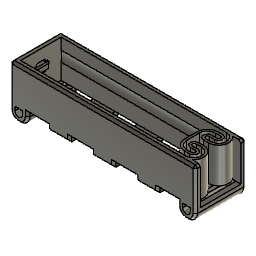
porta_pila_reforzado v2 (Autodesk Fusion 360 design; units mm, degrees)
Autodesk Fusion 360 part; units mm, degrees
note: some values were not read from the file. Set by a fixed rule: which face or edge a step refers to.
sketch "Sketch1" plane through (0, 0, 0) normal (0, 0, 1) x (1, 0, 0)
  line L0 (42, -11.5) -> (-42, -11.5)
  line L1 (-42, -11.5) -> (-42, 11.5)
  line L2 (-42, 11.5) -> (42, 11.5)
  line L3 (42, 11.5) -> (42, -11.5)
  line L4 (42, -11.5) -> (-42, 11.5) construction
  line L5 (-42, -11.5) -> (42, 11.5) construction
  dimension "d1" = 23
  dimension "d2" = 84
  constraint perpendicular L0 L1
  constraint parallel L0 L2
  constraint parallel L1 L3
  constraint horizontal L0
  constraint coincident L4 origin
  constraint coincident L5 origin
  measures "d1" distance of L0.end L1.end
  measures "d2" distance of L1.end L2.end
  measures "d8" distance of L0.start
extrude "Extrude1" add sketch "Sketch1" along normal blind 17
sketch "Sketch2" plane through (0, 0, 17) normal (0, 0, 1) x (-1, 0, 0)
  line L0 (-42, -11.5) -> (42, -11.5)
  line L1 (42, -11.5) -> (42, 11.5)
  line L2 (42, 11.5) -> (-42, 11.5)
  line L3 (-42, 11.5) -> (-42, -11.5)
  line L4 (39.5, -9.2) -> (-28.5, -9.2)
  line L5 (-28.5, -9.2) -> (-28.5, 9.2)
  line L6 (-28.5, 9.2) -> (39.5, 9.2)
  line L7 (39.5, 9.2) -> (39.5, -9.2)
  line L8 (42, 0) -> (39.5, 0) construction
  dimension "d5" = 68
  dimension "d6" = 18.4
  dimension "d7" = 2.5
  dimension "d8" = 1.8
  constraint horizontal L4
  constraint vertical L5
  constraint horizontal L6
  constraint vertical L7
  constraint midpoint L1 L8.start
  constraint midpoint L7 L8.end
  constraint horizontal L8
  measures "d5" distance of L4.start L4.end
  measures "d6" distance of L4.start L6.end
  measures "d7" distance of L1 L7
extrude "Extrude2" cut sketch "Sketch2" against normal through all contours L4 L5 L6 L7
sketch "Sketch3" plane through (28.5, 0, 0) normal (-1, 0, 0) x (0, -1, 0)
  line L0 (-9.2, 0) -> (9.2, 0)
  line L1 (9.2, 0) -> (9.2, 17)
  line L2 (9.2, 17) -> (-9.2, 17)
  line L3 (-9.2, 17) -> (-9.2, 0)
  circle A0 centre (0, 9.5) radius 9.5
  dimension "d10" = 19
  constraint coincident origin A0
  constraint vertical origin A0.centre
  measures "d10" diameter of A0
extrude "Extrude3" cut sketch "Sketch3" along normal blind 68 contours L3 A0 | L1 A0
sketch "Sketch4" plane through (0, 0, 17) normal (0, 0, 1) x (-1, 0, 0)
  line L0 (39.5, 9.2) -> (39.5, -9.2)
  line L1 (39.5, -9.2) -> (-28.5, -9.2)
  line L2 (-28.5, -9.2) -> (-28.5, 9.2)
  line L3 (-28.5, 9.2) -> (39.5, 9.2)
  line L4 (-42, -11.5) -> (42, -11.5)
  line L5 (42, -11.5) -> (42, 11.5)
  line L6 (42, 11.5) -> (-42, 11.5)
  line L7 (-42, 11.5) -> (-42, -11.5)
  line L8 (-28.5, 2.95) -> (-28.5, -2.95)
  arc A0 (-33.05, -7.5) -> (-28.5, -2.95) centre (-33.05, -2.95) ccw
  line L9 (-33.05, -7.5) -> (-35.45, -7.5)
  arc A1 (-35.45, -3.8) -> (-35.45, -7.5) centre (-35.45, -5.65) ccw
  line L10 (-35.45, -3.8) -> (-33.05, -3.8)
  arc A2 (-33.05, -3.8) -> (-33.05, -2.1) centre (-33.05, -2.95) ccw
  line L11 (-33.05, -2.1) -> (-35.45, -2.1)
  arc A3 (-35.45, -2.1) -> (-35.45, -9.2) centre (-35.45, -5.65) ccw
  line L12 (-35.45, -9.2) -> (-28.5, -9.2)
  line L13 (-35.45, -10.2) -> (-28.5, -10.2)
  arc A4 (-35.45, -1.1) -> (-35.45, -10.2) centre (-35.45, -5.65) ccw
  line L14 (-33.05, -1.1) -> (-35.45, -1.1)
  arc A5 (-33.05, -4.8) -> (-33.05, -1.1) centre (-33.05, -2.95) ccw
  line L15 (-35.45, -4.8) -> (-33.05, -4.8)
  arc A6 (-35.45, -4.8) -> (-35.45, -6.5) centre (-35.45, -5.65) ccw
  line L16 (-33.05, -6.5) -> (-35.45, -6.5)
  arc A7 (-33.05, -6.5) -> (-29.5, -2.95) centre (-33.05, -2.95) ccw
  line L17 (-29.5, 2.95) -> (-29.5, -2.95)
  line L18 (-39, -11.5) -> (-39, 11.5) construction
  line L19 (-28.5, 0) -> (-42, 0)
  line L20 (-28.5, -9.2) -> (-28.5, -10.2)
  line L21 (-29.5, 2.95) -> (-28.5, 2.95)
  line L22 (-35.45, -10.2) -> (-42, -10.2)
  line L23 (-35.45, -9.2) -> (-42, -9.2)
  dimension "d14" = 3
  dimension "d20" = 1.7
  dimension "d21" = 1.7
  dimension "d22" = 1.5
  dimension "d23" = 1
  constraint tangent L8 A0
  constraint tangent A0 L9
  constraint tangent L9 A1
  constraint tangent A1 L10
  constraint tangent L10 A2
  constraint horizontal L11
  constraint tangent L11 A3
  constraint coincident L1.end L2.start
  constraint coincident A1.centre A3.centre
  constraint midpoint L2 L8
  constraint tangent A2 L11
  constraint tangent A3 L12
  constraint horizontal L12
  constraint horizontal L9
  constraint horizontal L10
  constraint coincident L4 L18.start
  constraint coincident L6 L18.end
  constraint perpendicular L6 L18
  constraint tangent A3 L18
  constraint parallel L12 L13
  constraint concentric A3 A4
  constraint parallel L11 L14
  constraint concentric A2 A5
  constraint parallel L10 L15
  constraint concentric A1 A6
  constraint parallel L9 L16
  constraint concentric A0 A7
  constraint parallel L8 L17
  constraint tangent L16 A7
  constraint tangent L13 A4
  constraint tangent L15 A6
  constraint tangent A4 L14
  constraint tangent L14 A5
  constraint tangent A5 L15
  constraint tangent A6 L16
  constraint tangent A7 L17
  constraint vertical L8
  constraint coincident A0.centre A2.centre
  constraint midpoint L8 L19.start
  constraint midpoint L7 L19.end
  constraint perpendicular L13 L20
  constraint horizontal L21
  constraint coincident L7 L22.end
  constraint tangent A4 L22
  constraint coincident L7 L23.end
  constraint tangent A3 L23
  measures "d14" distance of L7 L18
  measures "d20" distance of L9 L12
  measures "d21" distance of L15 L16
  measures "d23" distance of L12 L13
extrude "Extrude4" cut sketch "Sketch4" against normal through all contours L2 A0 L9 A1 L10 A2 L11 A3 L12 | L7 A4 L14 A5 L15 A6 L16 A7 L17 L19 L23
mirror "Mirror1" about plane through (0, 0, 0) normal (0, 1, 0) of "Extrude4"
extrude "Extrude5" cut 2 faces at (28.5, 9.2749, 9.8979) (28.5, -9.2749, 9.1021) along direction (1, 0, 0) blind 7.95
sketch "Sketch5" plane through (0, -11.5, 0) normal (0, -1, 0) x (1, 0, 0)
  line L0 (-42, 0) -> (42, 0)
  line L1 (42, 0) -> (42, 17)
  line L2 (42, 17) -> (-42, 17)
  line L3 (-42, 17) -> (-42, 0)
  circle A0 centre (-38, -1.7) radius 1.7
  circle A1 centre (38, -1.7) radius 1.7
  line L4 (-42, 0) -> (-42, -1.7)
  arc A2 (-42, -1.7) -> (-34, -1.7) centre (-38, -1.7) ccw
  line L5 (-34, -1.7) -> (-34, 0)
  line L6 (42, 0) -> (42, -1.7)
  arc A3 (34, -1.7) -> (42, -1.7) centre (38, -1.7) ccw
  line L7 (34, -1.7) -> (34, 0)
  line L8 (-36.3, -1.7) -> (-36.3, 0)
  line L9 (-39.7, -1.7) -> (-39.7, 0)
  line L10 (36.3, -1.7) -> (36.3, 0)
  line L11 (39.7, -1.7) -> (39.7, 0)
  dimension "d29" = 3.4
  dimension "d30" = 2.3
  dimension "d31" = 2.3
  dimension "d66" = 8.4
  constraint tangent L0 A0
  constraint tangent L0 A1
  constraint equal A0 A1
  constraint coincident L0.start L3.end
  constraint perpendicular L0 L4
  constraint tangent L4 A2
  constraint coincident L0 L5.end
  constraint perpendicular L0 L5
  constraint coincident A0.centre A2.centre
  constraint tangent A2 L5
  constraint coincident L0.end L1.start
  constraint perpendicular L0 L6
  constraint tangent L6 A3
  constraint coincident L0 L7.end
  constraint perpendicular L0 L7
  constraint coincident A1.centre A3.centre
  constraint tangent A3 L7
  constraint coincident A0 L8.start
  constraint coincident L0 L8.end
  constraint tangent A0 L8
  constraint perpendicular L0 L8
  constraint coincident A0 L9.start
  constraint coincident L0 L9.end
  constraint tangent A0 L9
  constraint perpendicular L0 L9
  constraint coincident A1 L10.start
  constraint coincident L0 L10.end
  constraint tangent A1 L10
  constraint perpendicular L0 L10
  constraint coincident A1 L11.start
  constraint coincident L0 L11.end
  constraint tangent A1 L11
  constraint perpendicular L0 L11
  measures "d29" diameter of A0
  measures "d30" distance of A0 A2
  measures "d31" distance of A1 A3
extrude "Extrude6" add sketch "Sketch5" against normal blind 23 contours L0 A0 L4 A2 L5 L8 L9 | L0 A1 L6 A3 L7 L10 L11
sketch "Sketch7" plane through (42, 0, 0) normal (1, 0, 0) x (0, 1, 0)
  line L0 (-9.2, 17) -> (-11.5, 17)
  line L1 (-11.5, 17) -> (-11.5, -1.7)
  line L2 (-11.5, -1.7) -> (11.5, -1.7)
  line L3 (11.5, -1.7) -> (11.5, 17)
  line L4 (9.2, 0) -> (-9.2, 0)
  line L5 (-9.2, 0) -> (11.2, 0)
  line L6 (11.2, 0) -> (11.2, 1)
  line L7 (11.2, 1) -> (-9.2, 1)
  line L8 (-9.2, 1) -> (-9.2, 0)
  line L9 (-9.2, 0) -> (-9.2, 17)
  line L10 (11.5, 17) -> (9.2, 17)
  line L11 (9.2, 17) -> (9.2, 0)
  dimension "d39" = 1
  constraint horizontal L5
  constraint vertical L6
  constraint horizontal L7
  constraint vertical L8
  constraint coincident L4.end L5.start
  measures "d39" distance of L4.end L7.end
extrude "Extrude8" cut sketch "Sketch7" against normal blind 13.5 contours L4 L5 L7 L8 L9 L11 | L5 L6 L7 L11
extrude "Extrude14" add 2 faces at (28.5, 9.8667, 0.3333) (28.5, 9.8667, 0.3333) along direction (1, 0, 0) up to surface end surface through (42, 11.5, 0) normal (1, 0, 0) offset 0
sketch "Sketch8" plane through (28.5, 0, 0) normal (-1, 0, 0) x (0, -1, 0)
  line L0 (2.95, 1) -> (2.95, 17)
  line L1 (2.95, 17) -> (-2.95, 17)
  line L2 (-2.95, 17) -> (-2.95, 1)
  arc A0 (9.2, 7.1315) -> (9.2, 11.8685) centre (0, 9.5) ccw
  line L3 (2.95, 8) -> (-2.95, 8)
  line L4 (-2.95, 8) -> (-2.95, 11)
  line L5 (-2.95, 11) -> (2.95, 11)
  line L6 (2.95, 11) -> (2.95, 8)
  line L7 (2.95, 8) -> (-2.95, 11) construction
  line L8 (-2.95, 8) -> (2.95, 11) construction
  line L9 (-2.95, 1) -> (2.95, 1)
  point P0 (0, 9.5)
  dimension "d42" = 3
  constraint perpendicular L3 L4
  constraint parallel L3 L5
  constraint parallel L4 L6
  constraint horizontal L3
  constraint coincident L0 L3.start
  constraint coincident L7 P0
  constraint coincident L8 P0
  constraint coincident P0 A0.centre
  measures "d42" distance of L3.end L4.end
extrude "Extrude9" add sketch "Sketch8" along normal blind 1 contours L0 L2 L3 L4 L5 L6
fillet "Fillet1" radius 0.5 4 edges at (27.5, 0, 11) (27.5, 0, 8) (27.5, -2.95, 9.5) (27.5, 2.95, 9.5)
sketch "Sketch9" plane through (28.5, 0, 0) normal (-1, 0, 0) x (0, -1, 0)
  line L0 (-2.95, 11) -> (2.95, 11)
  line L1 (2.95, 11) -> (2.95, 17)
  line L2 (2.95, 17) -> (-2.95, 17)
  line L3 (-2.95, 17) -> (-2.95, 11)
  line L4 (-2, 12) -> (2, 12)
  line L5 (2, 12) -> (2, 11)
  line L6 (2, 11) -> (-2, 11)
  line L7 (-2, 11) -> (-2, 12)
  line L8 (-2, 7) -> (2, 7)
  line L9 (2, 7) -> (2, 8)
  line L10 (2, 8) -> (-2, 8)
  line L11 (-2, 8) -> (-2, 7)
  line L12 (-2.95, 8) -> (2.95, 8)
  dimension "d46" = 1
  dimension "d47" = 4
  dimension "d48" = 1
  dimension "d49" = 4
  constraint horizontal L4
  constraint vertical L5
  constraint horizontal L6
  constraint vertical L7
  constraint horizontal L8
  constraint vertical L9
  constraint horizontal L10
  constraint vertical L11
  constraint midpoint L10 L12
  constraint midpoint L0 L6
  measures "d46" distance of L4.start L6.end
  measures "d47" distance of L4.start L4.end
  measures "d48" distance of L8.start L10.end
  measures "d49" distance of L8.start L8.end
extrude "Extrude10" cut sketch "Sketch9" against normal blind 1 contours L0 L4 L5 L6 L7 | L8 L9 L10 L11 L12
sketch "Sketch10" plane through (-39.5, 0, 0) normal (1, 0, 0) x (0, 1, 0)
  arc A0 (-9.2, 11.8685) -> (-9.2, 7.1315) centre (0, 9.5) ccw
  line L0 (-9.2, 7.1315) -> (-9.2, 0)
  line L1 (9.2, 0) -> (9.2, 7.1315)
  arc A1 (9.2, 7.1315) -> (9.2, 11.8685) centre (0, 9.5) ccw
  line L2 (9.2, 11.8685) -> (9.2, 17)
  line L3 (9.2, 17) -> (-9.2, 17)
  line L4 (-9.2, 17) -> (-9.2, 11.8685)
  line L5 (3, 8) -> (-3, 8)
  line L6 (-3, 8) -> (-3, 11)
  line L7 (-3, 11) -> (3, 11)
  line L8 (3, 11) -> (3, 8)
  line L9 (3, 8) -> (-3, 11) construction
  line L10 (-3, 8) -> (3, 11) construction
  line L11 (-9.2, 0) -> (9.2, 0)
  point P0 (0, 9.5)
  dimension "d52" = 6
  dimension "d53" = 3
  constraint perpendicular L5 L6
  constraint parallel L5 L7
  constraint parallel L6 L8
  constraint horizontal L5
  constraint coincident L9 P0
  constraint coincident L10 P0
  constraint coincident P0 A0.centre
  measures "d52" distance of L6.end L7.end
  measures "d53" distance of L5.end L6.end
extrude "Extrude11" add sketch "Sketch10" along normal blind 1 contours L5 L6 L7 L8
fillet "Fillet2" radius 0.5 4 edges at (-38.5, 0, 11) (-38.5, 0, 8) (-38.5, 3, 9.5) (-38.5, -3, 9.5)
sketch "Sketch11" plane through (-39.5, 0, 0) normal (1, 0, 0) x (0, 1, 0)
  line L0 (3, 11) -> (3, 8)
  line L1 (3, 8) -> (-3, 8)
  line L2 (-3, 8) -> (-3, 11)
  line L3 (-3, 11) -> (3, 11)
  arc A0 (-9.2, 11.8685) -> (-9.2, 7.1315) centre (0, 9.5) ccw
  line L4 (-9.2, 7.1315) -> (-9.2, 0)
  line L5 (9.2, 0) -> (9.2, 7.1315)
  arc A1 (9.2, 7.1315) -> (9.2, 11.8685) centre (0, 9.5) ccw
  line L6 (9.2, 11.8685) -> (9.2, 17)
  line L7 (9.2, 17) -> (-9.2, 17)
  line L8 (-9.2, 17) -> (-9.2, 11.8685)
  line L9 (-2, 12) -> (2, 12)
  line L10 (2, 12) -> (2, 11)
  line L11 (2, 11) -> (-2, 11)
  line L12 (-2, 11) -> (-2, 12)
  line L13 (-2, 8) -> (2, 8)
  line L14 (2, 8) -> (2, 7)
  line L15 (2, 7) -> (-2, 7)
  line L16 (-2, 7) -> (-2, 8)
  line L17 (-9.2, 0) -> (9.2, 0)
  dimension "d57" = 4
  dimension "d58" = 1
  dimension "d59" = 4
  dimension "d60" = 1
  constraint horizontal L9
  constraint vertical L10
  constraint horizontal L11
  constraint vertical L12
  constraint horizontal L13
  constraint vertical L14
  constraint horizontal L15
  constraint vertical L16
  constraint midpoint L3 L11
  constraint midpoint L1 L13
  measures "d57" distance of L9.start L9.end
  measures "d58" distance of L9.start L11.end
  measures "d59" distance of L13.start L13.end
  measures "d60" distance of L13.start L15.end
extrude "Extrude12" cut sketch "Sketch11" against normal through all contours L3 L9 L10 L11 L12 | L1 L13 L14 L15 L16
sketch "Sketch12" plane through (0, -11.5, 0) normal (0, -1, 0) x (1, 0, 0)
  line L0 (36.3, 0) -> (39.7, 0)
  line L1 (39.7, 0) -> (39.7, -1.7)
  arc A0 (36.3, -1.7) -> (39.7, -1.7) centre (38, -1.7) ccw
  line L2 (36.3, -1.7) -> (36.3, 0)
  line L3 (-39.7, 0) -> (-36.3, 0)
  line L4 (-36.3, 0) -> (-36.3, -1.7)
  arc A1 (-39.7, -1.7) -> (-36.3, -1.7) centre (-38, -1.7) ccw
  line L5 (-39.7, -1.7) -> (-39.7, 0)
  line L6 (34, 0) -> (34, -1.7)
  arc A2 (34, -1.7) -> (42, -1.7) centre (38, -1.7) ccw
  line L7 (42, -1.7) -> (42, 17)
  line L8 (42, 17) -> (-42, 17)
  line L9 (-42, 17) -> (-42, -1.7)
  arc A3 (-42, -1.7) -> (-34, -1.7) centre (-38, -1.7) ccw
  line L10 (-34, -1.7) -> (-34, 0)
  line L11 (-34, 0) -> (34, 0)
  line L12 (-5, 0) -> (5, 0)
  line L13 (5, 0) -> (5, -2)
  line L14 (5, -2) -> (-5, -2)
  line L15 (-5, -2) -> (-5, 0)
  dimension "d62" = 10
  dimension "d63" = 2
  constraint horizontal L12
  constraint vertical L13
  constraint horizontal L14
  constraint vertical L15
  constraint midpoint origin L12
  measures "d62" distance of L12.start L12.end
  measures "d63" distance of L12.start L14.end
extrude "Extrude13" add sketch "Sketch12" against normal blind 23 contours L11 L12 L13 L14 L15
pattern_linear "R-Pattern1" count 3 spacing 20 along (1, 0, 0) both ways of "Extrude13"
chamfer "Chamfer1" distance 1 angle 45 43 edges at (0, -11.5, 17) (42, -10.35, 17) (34, -11.5, -0.85) (38, -11.5, -5.7) (42, -11.5, 7.65) (29.5, -11.5, 0) (25, -11.5, -1) (20, -11.5, -2) (15, -11.5, -1) (10, -11.5, 0) (5, -11.5, -1) (0, -11.5, -2) (-5, -11.5, -1) (-10, -11.5, 0) (-15, -11.5, -1) (-20, -11.5, -2) (-25, -11.5, -1) (-29.5, -11.5, 0) (-42, -11.5, 7.65) (-38, -11.5, -5.7) (-34, -11.5, -0.85) (-42, 0, 17) (-34, 11.5, -0.85) (-38, 11.5, -5.7) (-42, 11.5, 7.65) (-29.5, 11.5, 0) (-20, 11.5, -2) (-25, 11.5, -1) (-15, 11.5, -1) (-10, 11.5, 0) (-5, 11.5, -1) (0, 11.5, -2) (5, 11.5, -1) (10, 11.5, 0) (15, 11.5, -1) (20, 11.5, -2) (25, 11.5, -1) (29.5, 11.5, 0) (42, 11.5, 7.65) (38, 11.5, -5.7) (34, 11.5, -0.85) (42, 10.35, 17) (0, 11.5, 17)
equation "d10 = 18.4 mm + 0.6 mm"
